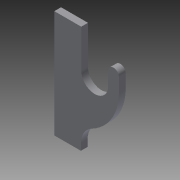
# Autodesk Inventor part: Can Hook
Saved by Autodesk Inventor 2015 (Build 190159000, 159)
## iProperties
Created: 2015-01-20
Part Number: Can Hook
Material: Generic
Document SubType Name: Modeling
Designer: nilesstanton
Density: 1 g/cm^3
Appearance: Default
Author: nilesstanton
Autodesk Inventor part; units mm, degrees
ref_plane "YZ Plane" through (0, 0, 0) normal (1, 0, 0) x (0, 1, 0)
ref_plane "XZ Plane" through (0, 0, 0) normal (0, 1, 0) x (-1, 0, 0)
ref_plane "XY Plane" through (0, 0, 0) normal (0, 0, 1) x (1, 0, 0)
sketch "Sketch1" plane through (0, 0, 0) normal (0, 0, 1) x (1, 0, 0)
  line L0 (0, 0) -> (0, 101.6)
  line L1 (0, 101.6) -> (25.4, 101.6)
  line L2 (25.4, 101.6) -> (25.4, 65.5898)
  line L3 (50.8, 65.5898) -> (50.8, 78.2898)
  line L4 (60.96, 78.2898) -> (60.96, 65.5898)
  line L5 (25.0337, 0) -> (0, 0)
  arc A0 (38.1, 52.8898) -> (50.8, 65.5898) centre (38.1, 65.5898) ccw
  arc A1 (25.4, 65.5898) -> (38.7011, 52.904) centre (38.1, 65.5898) ccw
  arc A2 (60.96, 78.2898) -> (50.8, 78.2898) centre (55.88, 78.2898) ccw
  line L6 (25.4, 65.5898) -> (50.8, 65.5898) construction
  arc A3 (35.4242, 23.2943) -> (60.96, 65.5898) centre (13.1646, 65.5898) ccw
  arc A4 (35.4242, 23.2943) -> (25.0337, 6.0842) centre (44.4817, 6.0842) ccw
  line L7 (25.0337, 6.0842) -> (25.0337, 0)
  dimension "d0" = 101.6
  dimension "d2" = 25.4
  dimension "d4" = 25.4
  dimension "d6" = 10.16
  dimension "d9" = 12.7
  dimension "d10" = 12.7
  dimension "d13" = 60.96
  constraints: 20 end point, 11 point on circle, 7 tangent, 5 centre point, 4 perpendicular, 3 parallel, 1 point on line, 1 vertical
  measures "d0" distance of L0.start L0.end
  measures "d2" distance of L0.end L1.end
  measures "d4" distance of L3.start L2.end
  measures "d6" distance of L3.end L4.start
  measures "d9" radius of A1
  measures "d10" distance of L3.start L3.end
  measures "d13" distance between parallel lines of L4 L0
extrude "Extrusion1" add sketch "Sketch1" along normal blind 6.35
body "Solid1"
